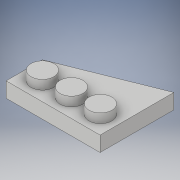
# Autodesk Inventor part: 3x1 diagonal
Saved by Autodesk Inventor 2017 (Build 210142000, 142)
## iProperties
Created: 2018-05-17
Part Number: 3x1 diagonal
Material: Generic
Document SubType Name: Modeling
Designer: 20000650
Density: 1 g/cm^3
Appearance: Default
Author: 20000650
Autodesk Inventor part; units mm, degrees
ref_plane "YZ Plane" through (0, 0, 0) normal (1, 0, 0) x (0, 1, 0)
ref_plane "XZ Plane" through (0, 0, 0) normal (0, 1, 0) x (-1, 0, 0)
ref_plane "XY Plane" through (0, 0, 0) normal (0, 0, 1) x (1, 0, 0)
sketch "Sketch1" plane through (0, 0, 0) normal (0, 1, 0) x (-1, 0, 0)
  line L0 (0, 0) -> (20.1574, 0)
  line L1 (20.1574, 0) -> (20.1574, -7.7978)
  line L2 (0, 0) -> (0, -15.8369)
  line L3 (0, -15.8369) -> (20.1574, -7.7978)
  dimension "d0" = 20.1574
  dimension "d1" = 7.7978
  dimension "d2" = 15.8369
  constraints: 8 end point, 1 horizontal, 1 perpendicular, 1 vertical
  measures "d0" distance of L0.start L0.end
  measures "d1" distance of L0.end L1.end
  measures "d2" distance of L0.start L2.end
extrude "Extrusion1" add sketch "Sketch1" along normal blind 3.236
sketch "Sketch2" plane through (0, 3.236, 0) normal (0, 1, 0) x (1, 0, 0)
  line L0 (0, 15.8369) -> (-20.1574, 7.7978) projected
  line L1 (0, 0) -> (0, 15.8369) projected
  line L2 (-20.1574, 0) -> (-12.3596, 0)
  line L3 (-20.1574, 7.7978) -> (-20.1574, 0) projected
  circle A0 centre (-16.2585, 3.8989) radius 2.4498
  dimension "d6" = 4.8997
  constraints: 2 end point, 1 centre point, 1 horizontal
  measures "d6" diameter of A0
extrude "Extrusion2" add sketch "Sketch2" along normal blind 1.9837
pattern_linear "Rectangular Pattern1" count 3 spacing 6.223 along (1, 0, 0) of "Extrusion2"
body "Solid1"
